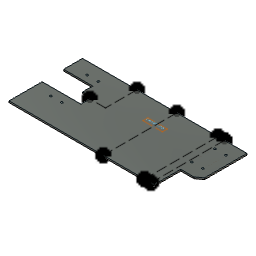
Metal Board v11 (Autodesk Fusion 360 design; units mm, degrees)
Autodesk Fusion 360 part; units mm, degrees
note: some values were not read from the file. Set by a fixed rule: which sketch regions a step uses.
sketch "Sketch1" plane through (0, 0, 0) normal (0, 0, 1) x (1, 0, 0)
  line L0 (0, 0) -> (680, 0)
  line L1 (680, 0) -> (680, -304)
  line L2 (680, -304) -> (0, -304)
  line L3 (0, -304) -> (0, 0)
  dimension "d1" = 680
  dimension "d2" = 304
  constraint horizontal L0
  constraint vertical L1
  constraint horizontal L2
  constraint vertical L3
  constraint coincident L0.start L3.end
  measures "d1" distance of L0.start L0.end
  measures "d2" distance of L0.start L2.end
extrude "Extrude1" add sketch "Sketch1" along normal blind 6.25
sketch "Sketch2" plane through (0, 0, 6.25) normal (0, 0, 1) x (-1, 0, 0)
  line L0 (0, 304) -> (-680, 304)
  line L1 (-680, 304) -> (-680, 0)
  line L2 (-680, 0) -> (0, 0)
  line L3 (0, 0) -> (0, 304)
  line L4 (-160, 120) -> (-160, 167)
  line L5 (-160, 167) -> (0, 167)
  line L6 (0, 167) -> (0, 78)
  line L7 (-120, 78) -> (-120, 120)
  line L8 (-120, 120) -> (-160, 120)
  line L9 (-120, 78) -> (0, 78)
  line L10 (-680, 304) -> (-600, 304)
  line L11 (-600, 304) -> (-600, 194)
  line L12 (-600, 194) -> (-655, 194)
  line L13 (-680, 175) -> (-680, 304)
  line L14 (-655, 194) -> (-680, 175)
  dimension "d10" = 120
  dimension "d11" = 42
  dimension "d12" = 47
  dimension "d13" = 120
  dimension "d14" = 160
  dimension "d15" = 110
  dimension "d19" = 129
  dimension "d20" = 55
  dimension "d21" = 80
  constraint vertical L4
  constraint horizontal L5
  constraint coincident L3 L6.end
  constraint perpendicular L5 L6
  constraint perpendicular L5 L7
  constraint perpendicular L7 L8
  constraint coincident L4.start L8.end
  constraint perpendicular L6 L9
  constraint horizontal L10
  constraint vertical L11
  constraint horizontal L12
  constraint vertical L13
  constraint coincident L0.end L1.start
  measures "d10" distance of L6.end L7.start
  measures "d11" distance of L7.start L7.end
  measures "d12" distance of L4.start L4.end
  measures "d13" distance of L2 L8
  measures "d14" distance of L4.end L5.end
  measures "d15" distance of L10.end L11.end
  measures "d19" distance of L0.end L13.start
  measures "d20" distance of L11.end L12.end
  measures "d21" distance of L0.end L10.end
extrude "Extrude3" cut sketch "Sketch2" against normal blind 6.25 contours L0 L1 L10 L11 L12 L13 L14 | L3 L4 L5 L6 L7 L8 L9
sketch "Sketch4" plane through (0, 0, 6.25) normal (0, 0, 1) x (-1, 0, 0)
  line L0 (-160, 167) -> (0, 167)
  line L1 (0, 167) -> (0, 304)
  line L2 (0, 304) -> (-600, 304)
  line L3 (-600, 304) -> (-600, 194)
  line L4 (-600, 194) -> (-655, 194)
  line L5 (-655, 194) -> (-680, 175)
  line L6 (-680, 175) -> (-680, 0)
  line L7 (-680, 0) -> (0, 0)
  line L8 (0, 0) -> (0, 78)
  line L9 (0, 78) -> (-120, 78)
  line L10 (-120, 78) -> (-120, 120)
  line L11 (-120, 120) -> (-160, 120)
  line L12 (-160, 120) -> (-160, 167)
  line L13 (-69, 200) -> (-115, 200) construction
  line L14 (-597, 145) -> (-643, 145) construction
  line L15 (-115, 50) -> (-69, 50) construction
  line L16 (-597, 50) -> (-643, 50) construction
  point P0 (-643, 145)
  point P1 (-597, 145)
  point P2 (-115, 200)
  point P3 (-69, 200)
  point P4 (-115, 50)
  point P5 (-69, 50)
  point P6 (-597, 50)
  point P7 (-643, 50)
  dimension "d33" = 46
  dimension "d35" = 150
  dimension "d36" = 50
  dimension "d37" = 95
  dimension "d38" = 115
  dimension "d44" = 83
  constraint horizontal P2 P3
  constraint horizontal P0 P1
  constraint coincident P3 L13.start
  constraint coincident P2 L13.end
  constraint parallel L7 L13
  constraint coincident P1 L14.start
  constraint coincident P0 L14.end
  constraint equal L13 L14
  constraint horizontal P4 P5
  constraint horizontal P5 P6
  constraint horizontal P6 P7
  constraint vertical P1 P6
  constraint coincident P4 L15.start
  constraint coincident P5 L15.end
  constraint coincident P6 L16.start
  constraint coincident P7 L16.end
  constraint equal L14 L16
  constraint equal L13 L15
  constraint vertical P2 P4
  constraint collinear L15 L16
  measures "d33" distance of P6 P7
  measures "d35" distance of P2 P4
  measures "d36" distance of L7 P4
  measures "d37" distance of P1 P6
  measures "d38" distance of L8 P4
  measures "d44" distance of L6 P6
hole "Hole2" at (597, -145, 6.25) at (643, -145, 6.25) at (115, -200, 6.25) at (69, -200, 6.25) at (115, -50, 6.25) at (69, -50, 6.25) at (643, -50, 6.25) at (597, -50, 6.25) direction (0, 0, -1) diameter 8.5 depth 6.25 tip angle 118
sketch "Sketch5" plane through (0, 0, 6.25) normal (0, 0, 1) x (-1, 0, 0)
  circle A0 centre (-643, 50) radius 4.25
  circle A1 centre (-115, 50) radius 4.25
  circle A2 centre (-115, 200) radius 4.25
  circle A3 centre (-597, 145) radius 4.25
  circle A4 centre (-643, 145) radius 4.25
  circle A5 centre (-69, 200) radius 4.25
  circle A6 centre (-69, 50) radius 4.25
  circle A7 centre (-597, 50) radius 4.25
  line L0 (-160, 167) -> (0, 167)
  line L1 (0, 167) -> (0, 304)
  line L2 (0, 304) -> (-600, 304)
  line L3 (-600, 304) -> (-600, 194)
  line L4 (-600, 194) -> (-655, 194)
  line L5 (-655, 194) -> (-680, 175)
  line L6 (-680, 175) -> (-680, 0)
  line L7 (-680, 0) -> (0, 0)
  line L8 (0, 0) -> (0, 78)
  line L9 (0, 78) -> (-120, 78)
  line L10 (-120, 78) -> (-120, 120)
  line L11 (-120, 120) -> (-160, 120)
  line L12 (-160, 120) -> (-160, 167)
  line L13 (-225, 0) -> (-225, 130) construction
  line L14 (-587, 0) -> (-587, 304) construction
  line L15 (-390, 0) -> (-390, 304) construction
  line L16 (-225, 130) -> (-160, 130) construction
  line L17 (-347.9611, 97.8111) -> (-427.9611, 97.8111) construction
  line L18 (-427.9611, 97.8111) -> (-427.9611, 77.8111) construction
  line L19 (-427.9611, 77.8111) -> (-347.9611, 77.8111) construction
  line L20 (-347.9611, 77.8111) -> (-347.9611, 97.8111) construction
  line L21 (-560, 0) -> (-560, 304) construction
  dimension "d39" = 225
  dimension "d41" = 390
  dimension "d42" = 130
  dimension "d43" = 10
  dimension "d46" = 170
  dimension "d47" = 93
  constraint coincident L7 L13.start
  constraint perpendicular L2 L13
  constraint coincident L7 L14.start
  constraint coincident L2 L14.end
  constraint perpendicular L2 L14
  constraint coincident L7 L15.start
  constraint coincident L2 L15.end
  constraint perpendicular L2 L15
  constraint coincident L12 L16.end
  constraint perpendicular L12 L16
  constraint coincident L7 L21.start
  constraint coincident L2 L21.end
  constraint perpendicular L2 L21
  measures "d39" distance of L8 L13
  measures "d41" distance of L1 L15
  measures "d42" distance of L7 L16
  measures "d46" distance of L15 L21
  measures "d47" distance of L6 L14
equation "d19 = 304 mm - 175 mm"
